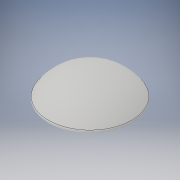
# Autodesk Inventor part: Button
Saved by Autodesk Inventor 2019 (Build 230136000, 136)
## iProperties
Created: 2019-02-14
Part Number: Button
Material: Generic
Document SubType Name: Modeling
Designer: lopez.xavier
Density: 1 g/cm^3
Appearance: Default
Author: lopez.xavier
Autodesk Inventor part; units mm, degrees
ref_plane "YZ Plane" through (0, 0, 0) normal (1, 0, 0) x (0, 1, 0)
ref_plane "XZ Plane" through (0, 0, 0) normal (0, 1, 0) x (-1, 0, 0)
ref_plane "XY Plane" through (0, 0, 0) normal (0, 0, 1) x (1, 0, 0)
sketch "Sketch1" plane through (0, 0, 0) normal (0, 0, 1) x (1, 0, 0)
  line L0 (0, 0) -> (25.4, 0)
  arc A0 (12.7, 7.62) -> (0, 0) centre (12.7, -6.7733) ccw
  arc A1 (25.4, 0) -> (12.7, 7.62) centre (12.7, -6.7733) ccw
  line L1 (12.7, 7.62) -> (4.6641, 7.62)
  line L2 (12.7, 7.62) -> (12.7, 0)
  dimension "d0" = 25.4
  dimension "d1" = 7.62
  dimension "d2" = 12.7
  constraints: 6 end point, 4 point on circle, 2 centre point, 2 horizontal, 2 tangent, 1 midpoint
  measures "d0" distance of L0.start L0.end
  measures "d1" distance from line of L0 L1.start
  measures "d2" horizontal distance of L0.end L1.start
revolve "Revolution1" add sketch "Sketch1" angle 360 about axis through (12.7, 7.62, 0) along (0, -1, 0) contours L2 A1 L0
fillet "Fillet1" radius 0.635 1 edges at (0, 0, 0)
sketch "Sketch2" plane through (12.7, 0, 0) normal (0, -1, 0) x (1, 0, 0)
  circle A0 centre (0, 0) radius 3.175
  circle A1 centre (0, 0) radius 11.5935 projected
  point P0 (-12.7, 0)
  dimension "d5" = 6.35
  dimension "d6" = 0
  constraints: 1 centre point
  measures "d5" diameter of A0
  measures "d6" distance of A1.centre A0.centre
extrude "Extrusion1" add sketch "Sketch2" along normal blind 2.54 contours A0
body "Solid1"
